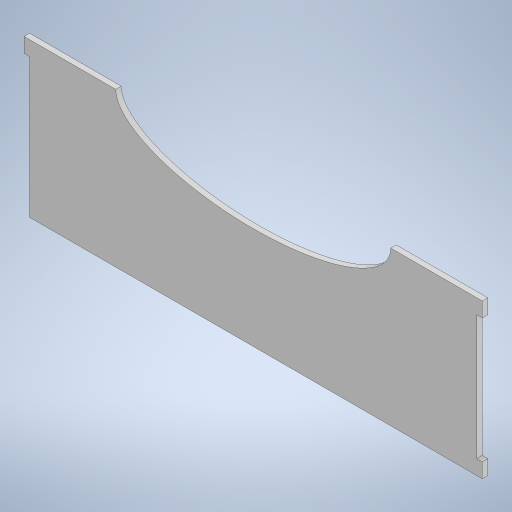
# Autodesk Inventor part: боковая стенка
Saved by Autodesk Inventor 2024.2 (Build 282272000, 272)
## iProperties
Created: 2025-11-20
Part Number: боковая стенка
Material: Типовые
Document SubType Name: Modeling
Designer: Zakhar
Density: 1 g/cm^3
Appearance: По умолчанию
Author: Zakhar
Autodesk Inventor part; units mm, degrees
ref_plane "YZ Plane" through (0, 0, 0) normal (1, 0, 0) x (0, 1, 0)
ref_plane "XZ Plane" through (0, 0, 0) normal (0, 1, 0) x (-1, 0, 0)
ref_plane "XY Plane" through (0, 0, 0) normal (0, 0, 1) x (1, 0, 0)
sketch "Эскиз1" plane through (0, 0, 0) normal (0, 0, 1) x (1, 0, 0)
  line L0 (127.4522, 43.2469) -> (127.4522, -40.7531)
  line L1 (127.4522, -40.7531) -> (-122.5478, -40.7531)
  line L2 (-122.5478, -40.7531) -> (-122.5478, 43.2469)
  line L3 (-119.5478, -40.7531) -> (-122.5478, -40.7531)
  line L4 (-119.5478, 35.2469) -> (-122.5478, 35.2469)
  line L5 (-119.5478, -40.7531) -> (-119.5478, -32.7531)
  line L6 (-122.5478, 35.2469) -> (-119.5478, 35.2469)
  line L7 (-119.5478, 35.2469) -> (-119.5478, -32.7531)
  line L8 (-119.5478, -32.7531) -> (-122.5478, -32.7531)
  line L9 (-122.5478, -32.7531) -> (-122.5478, 35.2469)
  ellipse E0 centre (2.4522, 43.2469) end of major axis (77.4522, 43.2469) minor radius 28.3094 (-72.5478, 43.2469) -> (77.4522, 43.2469) ccw
  line L10 (-122.5478, 43.2469) -> (-72.5478, 43.2469)
  line L11 (77.4522, 43.2469) -> (127.4522, 43.2469)
  line L12 (127.4522, 35.2469) -> (124.4522, 35.2469)
  line L13 (124.4522, 35.2469) -> (124.4522, -32.7531)
  line L14 (124.4522, -32.7531) -> (127.4522, -32.7531)
  line L15 (127.4522, -32.7531) -> (127.4522, 35.2469)
  point P0 (0, 0)
  point P1 (125.9522, -32.7531)
  dimension "d1" = 75
  dimension "d0" = 250
  dimension "d2" = 125
  dimension "d3" = 84
  dimension "d4" = 150
  dimension "d5" = 84
  dimension "d6" = 3
  dimension "d7" = 8
  constraints: 32 end point, 7 parallel, 4 horizontal, 4 perpendicular, 1 collinear, 1 midpoint, 1 point on line, 4 other
  measures "d0" distance of L1.start L1.end
  measures "d2" distance of L0.start point (2.452, 43.247)
  measures "d3" distance between parallel lines of L1 L11
  measures "d4" distance of L10.end L11.start
  measures "d5" distance from line of L1 point (2.452, 43.247)
  measures "d6" distance of L15.end L13.start
  measures "d7" vertical distance of point (125.952, -32.753) L1.start
extrude "Выдавливание1" add sketch "Эскиз1" along normal blind 3 contours L0 L12 L13 L14 L1 L5 L7 L4 L2 L10 E0 L11
